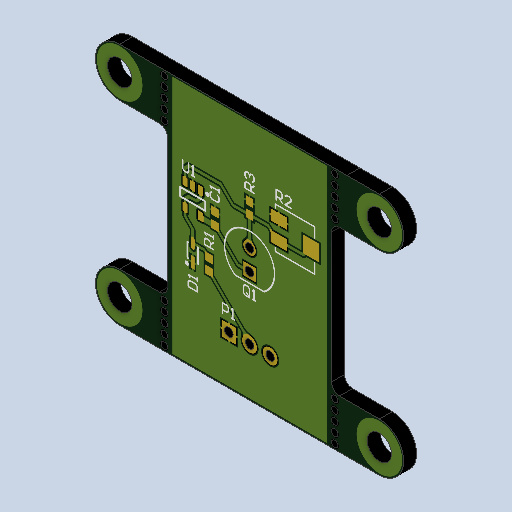
# Autodesk Inventor part: Dual PMT Controller - Light Interlock_BOARD
Saved by Autodesk Inventor 2023 (Build 270158000, 158)
## iProperties
Created: 2023-11-16
Part Number: Dual PMT Controller - Light Interlock_BOARD
Material: Generic
Document SubType Name: Modeling
Designer: Graeme
Density: 1 g/cm^3
Appearance: BoardColor
Author: Graeme
Autodesk Inventor part; units mm, degrees
ref_plane "YZ Plane" through (0, 0, 0) normal (1, 0, 0) x (0, 1, 0)
ref_plane "XZ Plane" through (0, 0, 0) normal (0, 1, 0) x (-1, 0, 0)
ref_plane "BoardFrontPlane" through (0, 0, 0) normal (0, 0, 1) x (1, 0, 0)
sketch "Sketch1" plane through (0, 0, 0) normal (0, 0, 1) x (1, 0, 0)
  line L0 (19.5, 24.465) -> (47.5, 24.465)
  line L1 (47.5, 24.465) -> (51.5, 24.465)
  arc A0 (51.5, 24.465) -> (51.5, 30.465) centre (51.5, 27.465) ccw
  line L2 (51.5, 30.465) -> (46.6, 30.4645)
  arc A1 (45.5997, 31.4679) -> (46.6, 30.4645) centre (46.6001, 31.4649) ccw
  line L3 (45.5997, 31.4679) -> (45.6001, 47.4621)
  arc A2 (46.6004, 48.4653) -> (45.6001, 47.4621) centre (46.6004, 47.465) ccw
  line L4 (46.6004, 48.4653) -> (51.5004, 48.465)
  arc A3 (51.5004, 48.465) -> (51.5004, 54.465) centre (51.5004, 51.465) ccw
  line L5 (51.5004, 54.465) -> (47.5004, 54.465)
  line L6 (47.5004, 54.465) -> (19.5004, 54.465)
  arc A4 (19.5004, 54.465) -> (19.5004, 48.465) centre (19.5004, 51.465) ccw
  line L7 (19.5004, 48.465) -> (24.4004, 48.4655)
  arc A5 (25.4007, 47.4621) -> (24.4004, 48.4655) centre (24.4003, 47.4651) ccw
  line L8 (25.4007, 47.4621) -> (25.4003, 31.4679)
  arc A6 (24.4, 30.4647) -> (25.4003, 31.4679) centre (24.4, 31.465) ccw
  line L9 (24.4, 30.4647) -> (19.5, 30.465)
  arc A7 (19.5, 30.465) -> (19.5, 24.465) centre (19.5, 27.465) ccw
  constraints: 20 end point, 16 point on circle, 8 centre point
extrude "BoardOutline" add sketch "Sketch1" along normal blind 1.5954
sketch "img_Top" plane through (0, 0, 1.5954) normal (0, 0, 1) x (1, 0, 0)
  line L0 (16.5, 54.465) -> (54.5017, 54.465) construction
  line L1 (54.5017, 54.465) -> (54.5017, 24.465) construction
  line L2 (54.5017, 24.465) -> (16.5, 24.465) construction
  line L3 (16.5, 24.465) -> (16.5, 54.465) construction
  constraints: 2 other
decal "Decal_Top"
sketch "img_Bottom" plane through (0, 0, -1.5954) normal (0, 0, -1) x (1, 0, 0)
  line L0 (16.5, -24.465) -> (54.5017, -24.465) construction
  line L1 (54.5017, -24.465) -> (54.5017, -54.465) construction
  line L2 (54.5017, -54.465) -> (16.5, -54.465) construction
  line L3 (16.5, -54.465) -> (16.5, -24.465) construction
  constraints: 2 other
decal "Decal_Bottom"
sketch "Sketch4" plane through (0, 0, 1.5954) normal (0, 0, 1) x (1, 0, 0)
  point P0 (35.5, 40.735)
hole "Q1-2" at (35.5, 40.735, 1.5954) direction (0, 0, -1) diameter 1.016 end through all
sketch "Sketch5" plane through (0, 0, 1.5954) normal (0, 0, 1) x (1, 0, 0)
  point P0 (35.5, 38.195)
hole "Q1-1" at (35.5, 38.195, 1.5954) direction (0, 0, -1) diameter 1.016 end through all
sketch "Sketch6" plane through (0, 0, 1.5954) normal (0, 0, 1) x (1, 0, 0)
  point P0 (46.0004, 53.865)
hole "Free-6_WBTLOXPK" at (46.0004, 53.865, 1.5954) direction (0, 0, -1) diameter 0.8 end through all
sketch "Sketch7" plane through (0, 0, 1.5954) normal (0, 0, 1) x (1, 0, 0)
  point P0 (46.0004, 52.665)
hole "Free-5_XIOJIJXP" at (46.0004, 52.665, 1.5954) direction (0, 0, -1) diameter 0.8 end through all
sketch "Sketch8" plane through (0, 0, 1.5954) normal (0, 0, 1) x (1, 0, 0)
  point P0 (46.0004, 51.465)
hole "Free-4_DJTYKPAA" at (46.0004, 51.465, 1.5954) direction (0, 0, -1) diameter 0.8 end through all
sketch "Sketch9" plane through (0, 0, 1.5954) normal (0, 0, 1) x (1, 0, 0)
  point P0 (46.0004, 50.265)
hole "Free-3_AXXACNQN" at (46.0004, 50.265, 1.5954) direction (0, 0, -1) diameter 0.8 end through all
sketch "Sketch10" plane through (0, 0, 1.5954) normal (0, 0, 1) x (1, 0, 0)
  point P0 (46.0004, 49.065)
hole "Free-2_AOCKDCBY" at (46.0004, 49.065, 1.5954) direction (0, 0, -1) diameter 0.8 end through all
sketch "Sketch11" plane through (0, 0, 1.5954) normal (0, 0, 1) x (1, 0, 0)
  point P0 (51.5004, 51.465)
hole "Free-1_DASBMRFB" at (51.5004, 51.465, 1.5954) direction (0, 0, -1) diameter 3 end through all
sketch "Sketch12" plane through (0, 0, 1.5954) normal (0, 0, 1) x (1, 0, 0)
  point P0 (25.0004, 53.865)
hole "Free-6_NIMWPQYT" at (25.0004, 53.865, 1.5954) direction (0, 0, -1) diameter 0.8 end through all
sketch "Sketch13" plane through (0, 0, 1.5954) normal (0, 0, 1) x (1, 0, 0)
  point P0 (25.0004, 52.665)
hole "Free-5_XNHNLNST" at (25.0004, 52.665, 1.5954) direction (0, 0, -1) diameter 0.8 end through all
sketch "Sketch14" plane through (0, 0, 1.5954) normal (0, 0, 1) x (1, 0, 0)
  point P0 (25.0004, 51.465)
hole "Free-4_FETUHRKC" at (25.0004, 51.465, 1.5954) direction (0, 0, -1) diameter 0.8 end through all
sketch "Sketch15" plane through (0, 0, 1.5954) normal (0, 0, 1) x (1, 0, 0)
  point P0 (25.0004, 50.265)
hole "Free-3_DMTDOSJH" at (25.0004, 50.265, 1.5954) direction (0, 0, -1) diameter 0.8 end through all
sketch "Sketch16" plane through (0, 0, 1.5954) normal (0, 0, 1) x (1, 0, 0)
  point P0 (25.0004, 49.065)
hole "Free-2_TMPFYMJS" at (25.0004, 49.065, 1.5954) direction (0, 0, -1) diameter 0.8 end through all
sketch "Sketch17" plane through (0, 0, 1.5954) normal (0, 0, 1) x (1, 0, 0)
  point P0 (19.5004, 51.465)
hole "Free-1_WWOKCKJL" at (19.5004, 51.465, 1.5954) direction (0, 0, -1) diameter 3 end through all
sketch "Sketch18" plane through (0, 0, 1.5954) normal (0, 0, 1) x (1, 0, 0)
  point P0 (51.5, 27.465)
hole "Free-1_SGRFTGBA" at (51.5, 27.465, 1.5954) direction (0, 0, -1) diameter 3 end through all
sketch "Sketch19" plane through (0, 0, 1.5954) normal (0, 0, 1) x (1, 0, 0)
  point P0 (46, 29.865)
hole "Free-2_AUMGPVUD" at (46, 29.865, 1.5954) direction (0, 0, -1) diameter 0.8 end through all
sketch "Sketch20" plane through (0, 0, 1.5954) normal (0, 0, 1) x (1, 0, 0)
  point P0 (46, 28.665)
hole "Free-3_HPVJLOHR" at (46, 28.665, 1.5954) direction (0, 0, -1) diameter 0.8 end through all
sketch "Sketch21" plane through (0, 0, 1.5954) normal (0, 0, 1) x (1, 0, 0)
  point P0 (46, 27.465)
hole "Free-4_DQHIBCUL" at (46, 27.465, 1.5954) direction (0, 0, -1) diameter 0.8 end through all
sketch "Sketch22" plane through (0, 0, 1.5954) normal (0, 0, 1) x (1, 0, 0)
  point P0 (46, 26.265)
hole "Free-5_OUJHCFEU" at (46, 26.265, 1.5954) direction (0, 0, -1) diameter 0.8 end through all
sketch "Sketch23" plane through (0, 0, 1.5954) normal (0, 0, 1) x (1, 0, 0)
  point P0 (46, 25.065)
hole "Free-6_RFLYKSPV" at (46, 25.065, 1.5954) direction (0, 0, -1) diameter 0.8 end through all
sketch "Sketch24" plane through (0, 0, 1.5954) normal (0, 0, 1) x (1, 0, 0)
  point P0 (25, 25.065)
hole "Free-6_SWLXYYKK" at (25, 25.065, 1.5954) direction (0, 0, -1) diameter 0.8 end through all
sketch "Sketch25" plane through (0, 0, 1.5954) normal (0, 0, 1) x (1, 0, 0)
  point P0 (25, 26.265)
hole "Free-5_RJKXWDHV" at (25, 26.265, 1.5954) direction (0, 0, -1) diameter 0.8 end through all
sketch "Sketch26" plane through (0, 0, 1.5954) normal (0, 0, 1) x (1, 0, 0)
  point P0 (25, 27.465)
hole "Free-4_KOIALDYT" at (25, 27.465, 1.5954) direction (0, 0, -1) diameter 0.8 end through all
sketch "Sketch27" plane through (0, 0, 1.5954) normal (0, 0, 1) x (1, 0, 0)
  point P0 (25, 28.665)
hole "Free-3_NUADKFXF" at (25, 28.665, 1.5954) direction (0, 0, -1) diameter 0.8 end through all
sketch "Sketch28" plane through (0, 0, 1.5954) normal (0, 0, 1) x (1, 0, 0)
  point P0 (25, 29.865)
hole "Free-2_KKFAPUKC" at (25, 29.865, 1.5954) direction (0, 0, -1) diameter 0.8 end through all
sketch "Sketch29" plane through (0, 0, 1.5954) normal (0, 0, 1) x (1, 0, 0)
  point P0 (19.5, 27.465)
hole "Free-1_BKUUHACL" at (19.5, 27.465, 1.5954) direction (0, 0, -1) diameter 3 end through all
sketch "Sketch30" plane through (0, 0, 1.5954) normal (0, 0, 1) x (1, 0, 0)
  point P0 (32.96, 30.465)
hole "P1-1" at (32.96, 30.465, 1.5954) direction (0, 0, -1) diameter 1.04 end through all
sketch "Sketch31" plane through (0, 0, 1.5954) normal (0, 0, 1) x (1, 0, 0)
  point P0 (35.5, 30.465)
hole "P1-2" at (35.5, 30.465, 1.5954) direction (0, 0, -1) diameter 1.04 end through all
sketch "Sketch32" plane through (0, 0, 1.5954) normal (0, 0, 1) x (1, 0, 0)
  point P0 (38.04, 30.465)
hole "P1-3" at (38.04, 30.465, 1.5954) direction (0, 0, -1) diameter 1.04 end through all
body "Solid1"
